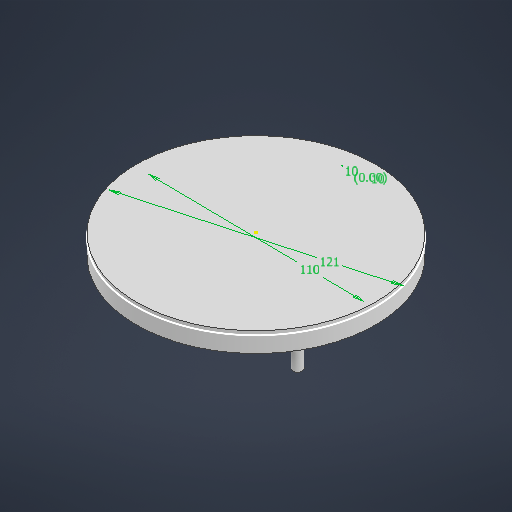
# Autodesk Inventor part: Cover
Saved by Autodesk Inventor 2026.2 (Build 302298000, 298)
## iProperties
Created: 2026-01-26
Part Number: Cover
Material: Generic
Document SubType Name: Modeling
Designer: Cobble
Density: 1 g/cm^3
Appearance: Default
Author: Cobble
Autodesk Inventor part; units mm, degrees
ref_plane "YZ Plane" through (0, 0, 0) normal (1, 0, 0) x (0, 1, 0)
ref_plane "XZ Plane" through (0, 0, 0) normal (0, 1, 0) x (-1, 0, 0)
ref_plane "XY Plane" through (0, 0, 0) normal (0, 0, 1) x (1, 0, 0)
sketch "Sketch1" plane through (0, 0, 0) normal (0, 0, 1) x (1, 0, 0)
  circle A0 centre (0, 0) radius 60.5
  circle A1 centre (0, 0) radius 55
  line L0 (0, 55) -> (-10, 55)
  line L1 (0, 55) -> (10, 55)
  line L2 (0, 55) -> (10, 55) construction
  line L3 (10, 59.6678) -> (10, 53.8845)
  line L4 (-10, 59.6678) -> (-10, 54.0833)
  point P0 (10, 54.0833)
  dimension "d0" = 121
  dimension "d1" = 110
  dimension "d45" = 10
  dimension "d46" = 10
  dimension "d47" = 0
  constraints: 10 end point, 5 point on circle, 3 horizontal, 2 centre point, 2 coincident, 2 tangent, 2 vertical, 1 collinear
  measures "d0" diameter of A0
  measures "d1" diameter of A1
  measures "d45" distance of L0.start L0.end
  measures "d46" distance of L1.start L1.end
  measures "d47" distance between parallel lines of L1 L2
extrude "Extrusion1" add sketch "Sketch1" along normal blind 2
extrude "Extrusion2" add sketch "Sketch1" against normal blind 8 contours A0 L4 A1 L3 | L3 L1 L0 L4 A0 | L3 A1 L1 | L0 A1 L4
sketch "Sketch11" plane through (0, 0, 0) normal (1, 0, 0) x (0, 1, 0)
  line L0 (60.5, 2) -> (-60.5, 2) projected
  line L1 (-60.5, -8) -> (60.5, -8) projected
  line L2 (59.6678, 0) -> (54.0833, 0) projected
  line L3 (59.6678, 0) -> (59.6678, -6) projected
  line L4 (54.0833, -6) -> (59.6678, -6) projected
  line L5 (54.0833, 0) -> (54.0833, -6) projected
  line L6 (-60.5, -8) -> (60.5, -8) projected
  line L7 (55, -8) -> (-55, -8) projected
  line L8 (-60.5, -8) -> (60.5, -8) projected
  line L9 (60.5, 0) -> (-60.5, 0) projected
  line L10 (-55, -8) -> (-61, -8)
  line L11 (-61, -8) -> (-61, 0)
  line L12 (-61, 0) -> (-55, 0)
  line L13 (-55, 0) -> (-55, -8)
  line L14 (-61, -8) -> (-55, 0)
  circle A0 centre (-58, -4) radius 2.1
  line L15 (-61, -8) -> (-67, -8)
  line L16 (-67, -8) -> (-67, -2)
  line L17 (-67, -2) -> (-61, -2)
  line L18 (-61, -2) -> (-61, -8)
  line L19 (-61, -8) -> (-67, -2)
  circle A1 centre (-64, -5) radius 2.15
  point P0 (0, 0)
  point P1 (42.0833, 0)
  point P2 (42.0833, -6)
  point P3 (48.0833, -6)
  dimension "d48" = 6
  dimension "d49" = 4.2
  dimension "d50" = 6
  dimension "d51" = 6
  dimension "d52" = 4.3
  constraints: 20 end point, 4 parallel, 2 centre point, 2 horizontal, 2 midpoint, 2 perpendicular, 1 point on line, 1 other
  measures "d48" distance of L11.end L12.end
  measures "d49" diameter of A0
  measures "d50" distance of L16.end L17.end
  measures "d51" distance of L15.end L16.end
  measures "d52" diameter of A1
sketch "Sketch12" plane through (0, 0, 2) normal (0, 0, 1) x (1, 0, 0)
  point P0 (0, 0)
sketch "Sketch13" plane through (0, 0, 0) normal (0, 1, 0) x (-1, 0, 0)
  line L0 (0, -6) -> (0, 2)
  line L1 (0, 0) -> (0, -1)
  line L2 (0, -1) -> (3.1, -1)
  line L3 (3.1, -1) -> (3.1, -7.2)
  line L4 (3.1, -7.2) -> (0, -7.2)
  line L5 (0, -7.2) -> (0, -1)
  line L6 (3.1, -7.2) -> (-3.1, -7.2)
  line L7 (-3.1, -7.2) -> (-3.1, -1)
  line L8 (-3.1, -1) -> (3.1, -1)
  line L9 (3.1, -1) -> (3.1, -7.2)
  line L10 (0, -4.1) -> (6, -4.1)
  line L11 (6, -4.1) -> (-6, -4.1)
  circle A0 centre (-6, -4.1) radius 2.15
  circle A1 centre (6, -4.1) radius 2.15
  point P0 (0, -7.2)
  dimension "d58" = 1
  dimension "d59" = 3.1
  dimension "d60" = 6.2
  dimension "d61" = 6.2
  dimension "d62" = 6.2
  dimension "d66" = 6
  dimension "d67" = 12
  dimension "d68" = 4.3
  dimension "d69" = 4.3
  constraints: 24 end point, 4 parallel, 3 horizontal, 2 centre point, 2 coincident, 2 perpendicular, 2 point on line, 1 midpoint
  measures "d58" distance of L1.start L1.end
  measures "d59" distance of L3.end L4.end
  measures "d60" distance of L2.end L3.end
  measures "d61" distance of L7.end L8.end
  measures "d62" distance of L6.end L7.end
  measures "d66" distance of L10.start L10.end
  measures "d67" distance of L10.end L11.end
  measures "d68" diameter of A0
  measures "d69" diameter of A1
extrude "Extrusion12" cut sketch "Sketch13" along normal through all
fillet "Fillet3" radius 0.3 4 edges at (-3.1, 57.6665, -1) (3.1, 57.6665, -1) (3.1, 57.6665, -7.2) (-3.1, 57.6665, -7.2)
sketch "Sketch14" plane through (0, 0, -8) normal (0, 0, -1) x (-1, 0, 0)
  circle A0 centre (0, 0) radius 57.5
  circle A1 centre (0, 57.5) radius 2.4
  circle A2 centre (-49.7965, -28.75) radius 2.4
  circle A3 centre (49.7965, -28.75) radius 2.4
  point P0 (50.9528, -26.6469)
  point P1 (48.5533, -30.803)
  dimension "d70" = 115
  dimension "d71" = 4.8
  dimension "d74" = 360
  constraints: 3 centre point, 1 coincident, 10 other
  measures "d71" diameter of A1
extrude "Extrusion13" add sketch "Sketch14" along normal blind 10 contours A1 A0 | A0 A1 | A0 A3 | A2 A0 | A0 A2 picked at (49.0578, -28.4334)
body "Solid1"
